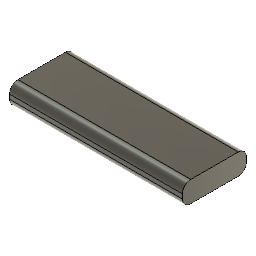
1570 100mAh Lipo Battery (Autodesk Fusion 360 design; units mm, degrees)
Autodesk Fusion 360 part; units mm, degrees
sketch "Sketch1" plane through (0, 0, 0) normal (0, 0, 1) x (1, 0, 0)
  line L0 (0, 0) -> (31, 0)
  line L1 (31, 0) -> (31, 11.5)
  line L2 (31, 11.5) -> (0, 11.5)
  line L3 (0, 11.5) -> (0, 0)
  dimension "d1" = 31
  dimension "d2" = 11.5
  measures "d1" distance of L0.start L0.end
  measures "d2" distance of L0.start L2.end
extrude "Extrude1" add sketch "Sketch1" along normal blind 3.8
fillet "Fillet1" radius 1.5 4 edges at (15.5, 0, 3.8) (15.5, 0, 0) (15.5, 11.5, 3.8) (15.5, 11.5, 0)
